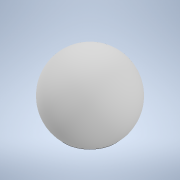
# Autodesk Inventor part: Ch7(5) Part 4 Ball End
Saved by Autodesk Inventor 2020 (Build 240168000, 168)
## iProperties
Created: 2021-03-04
Part Number: Ch7(5) Part 4 Ball End
Material: Generic
Document SubType Name: Modeling
Designer: adriggs
Density: 1 g/cm^3
Appearance: Default
Author: adriggs
Autodesk Inventor part; units mm, degrees
ref_plane "YZ Plane" through (0, 0, 0) normal (1, 0, 0) x (0, 1, 0)
ref_plane "XZ Plane" through (0, 0, 0) normal (0, 1, 0) x (-1, 0, 0)
ref_plane "XY Plane" through (0, 0, 0) normal (0, 0, 1) x (1, 0, 0)
sketch "Sketch1" plane through (0, 0, 0) normal (1, 0, 0) x (0, 1, 0)
  line L0 (-2.8185, 0) -> (16.9108, 0) projected
  line L1 (0, -11.8099) -> (0, 7.5246) projected
  arc A0 (0, -4.7625) -> (12.4535, 0) centre (5.3161, 0) ccw
  line L2 (0, 4.7625) -> (0, -4.7625)
  point P0 (0, 0)
  dimension "d1" = 14.2748
  dimension "d3" = 9.525
  constraints: 2 end point, 2 point on circle, 2 point on line, 1 centre point, 1 midpoint, 1 vertical
  measures "d1" diameter of A0
  measures "d3" distance of L2.end L2.start
revolve "Revolution1" add sketch "Sketch1" angle 360 about axis through (0, -10, 0) along (0, 1, 0)
sketch "Sketch2" plane through (0, 0, 0) normal (0, -1, 0) x (1, 0, 0)
  circle A0 centre (0, 0) radius 3.1623
  dimension "d5" = 6.3246
  constraints: 1 centre point, 1 coincident
  measures "d5" diameter of A0
extrude "Extrusion1" cut sketch "Sketch2" against normal blind 10.16
body "Solid1"
